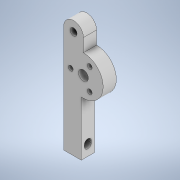
# Autodesk Inventor part: Motor_holder
Saved by Autodesk Inventor 2021 (Build 250183000, 183)
## iProperties
Created: 2024-05-11
Part Number: Motor_holder
Material: Generic
Document SubType Name: Modeling
Designer: Lukas
Density: 1 g/cm^3
Appearance: Default
Author: Lukas
Autodesk Inventor part; units mm, degrees
ref_plane "YZ Plane" through (0, 0, 0) normal (1, 0, 0) x (0, 1, 0)
ref_plane "XZ Plane" through (0, 0, 0) normal (0, 1, 0) x (-1, 0, 0)
ref_plane "XY Plane" through (0, 0, 0) normal (0, 0, 1) x (1, 0, 0)
sketch "Sketch1" plane through (0, 0, 0) normal (0, 0, 1) x (1, 0, 0)
  circle A0 centre (0, 0) radius 2.25
  circle A1 centre (-4.5, 15) radius 1.6
  circle A2 centre (-5.774, 0) radius 1.1
  circle A3 centre (2.8863, 5) radius 1.1
  circle A4 centre (2.8863, -5) radius 1.1
  line L0 (-1, -34) -> (-1, -9)
  line L1 (-1, -9) -> (0, -9)
  arc A5 (0, 15) -> (-9, 15) centre (-4.5, 15) ccw
  line L2 (0, 15) -> (0, 9)
  arc A6 (0, -9) -> (0, 9) centre (0, 0) ccw
  line L3 (-9, 15) -> (-9, -34)
  line L4 (-9, -34) -> (-1, -34)
  dimension "d0" = 10
  dimension "d1" = 10
  dimension "d2" = 10
  dimension "d3" = 5
  dimension "d4" = 5.774
  dimension "d5" = 3.2
  dimension "d6" = 9
  dimension "d7" = 9
  dimension "d8" = 15
  dimension "d9" = 25
  dimension "d10" = 8
  dimension "d11" = 2.2
  dimension "d12" = 4.5
  constraints: 10 end point, 7 centre point, 5 point on circle, 3 coincident, 3 tangent, 3 vertical, 2 equal radius, 2 perpendicular, 2 vertical alignment
  measures "d0" distance of A4.centre A3.centre
  measures "d1" distance of A2.centre A4.centre
  measures "d2" distance of A2.centre A3.centre
  measures "d3" vertical distance of A3.centre A0.centre
  measures "d4" distance of A2.centre A0.centre
  measures "d5" diameter of A1
  measures "d6" radius of A6
  measures "d7" distance between parallel lines of L3 L2
  measures "d8" vertical distance of A1.centre point (0, 0)
  measures "d9" distance from line of L0.end L4
  measures "d10" distance of L3.end L0.start
  measures "d11" diameter of A3
  measures "d12" diameter of A0
extrude "Extrusion1" add sketch "Sketch1" along normal blind 6
sketch "Sketch2" plane through (-9, -34, 0) normal (-1, 0, 0) x (0, 0, 1)
  line L0 (0, 0) -> (6, 0) projected
  line L1 (3, 4.6) -> (3, 5.4) construction
  line L2 (4.6, 4.6) -> (4.6, 5.4)
  line L3 (1.4, 5.4) -> (1.4, 4.6)
  arc A0 (1.4, 4.6) -> (4.6, 4.6) centre (3, 4.6) ccw
  arc A1 (4.6, 5.4) -> (1.4, 5.4) centre (3, 5.4) ccw
  point P0 (0, 34)
  point P1 (3, 5)
  point P2 (3, 0)
  dimension "d20" = 3.2
  dimension "d21" = 5
  dimension "d22" = 4
  constraints: 8 end point, 4 point on circle, 4 tangent, 2 centre point, 2 midpoint, 1 parallel, 1 vertical, 1 vertical alignment
  measures "d20" distance between parallel lines of L2 L3
  measures "d21" distance of point (3, 0) point (3, 5)
extrude "Extrusion2" cut sketch "Sketch2" against normal through all
sketch "Sketch3" plane through (0, 0, 0) normal (0, 0, -1) x (-1, 0, 0)
  circle A0 centre (5.774, 0) radius 1.1 projected
  circle A1 centre (5.774, 0) radius 1.1 projected
  circle A2 centre (-2.8863, -5) radius 1.1 projected
  circle A3 centre (-2.8863, -5) radius 1.1 projected
  circle A4 centre (-2.8863, 5) radius 1.1 projected
  circle A5 centre (-2.8863, 5) radius 1.1 projected
  circle A6 centre (5.774, 0) radius 2.25
  circle A7 centre (-2.8863, -5) radius 2.25
  circle A8 centre (-2.8863, 5) radius 2.25
  point P0 (0, 0)
  dimension "d25" = 4.5
  constraints: 3 centre point, 3 coincident, 2 equal radius
  measures "d25" diameter of A6
extrude "Extrusion3" cut sketch "Sketch3" against normal blind 3
equation "\"d1\" = d0"
equation "\"d2\" = d0"
equation "\"d3\" = 0.5 * d0"
body "Solid1"
